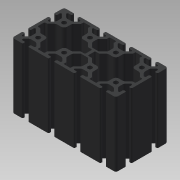
# Autodesk Inventor part: 40-8016
Saved by Autodesk Inventor 2013 (Build 170138000, 138)
## iProperties
Company: 80/20 Inc.
Created: 2014-04-23
Part Number: 40-8016
Material: Generic
Document SubType Name: Modeling
Designer: Ross Bowman
Density: 1 g/cm^3
Engineer: Ross Bowman
Catalog Web Link: 8020.net
Vendor: 80/20 Inc.
Material: 6105-T5 Aluminum
Author: Ross Bowman
Keywords: 80/20 , 8020 , T-Slot , Extrusion
Autodesk Inventor part; units mm, degrees
ref_plane "YZ Plane" through (0, 0, 0) normal (1, 0, 0) x (0, 1, 0)
ref_plane "XZ Plane" through (0, 0, 0) normal (0, 1, 0) x (-1, 0, 0)
ref_plane "XY Plane" through (0, 0, 0) normal (0, 0, 1) x (1, 0, 0)
sketch "Sketch1" plane through (0, 0, 0) normal (0, 0, 1) x (1, 0, 0)
  circle A0 centre (-19.8932, -20) radius 3.4
  circle A1 centre (-59.9459, -20) radius 3.4
  circle A2 centre (-59.9233, 20) radius 3.4
  line L0 (-29.0146, 25.9413) -> (-34.3182, 31.245)
  arc A3 (-27.6247, 22.586) -> (-29.0146, 25.9413) centre (-32.3699, 22.586) ccw
  line L1 (-27.6247, 16.9863) -> (-27.6247, 22.586)
  arc A4 (-27.6247, 16.9863) -> (-22.8702, 12.2331) centre (-22.8715, 16.9863) ccw
  line L2 (-17.2771, 12.2347) -> (-22.8702, 12.2331)
  arc A5 (-13.9164, 10.8432) -> (-17.2771, 12.2347) centre (-17.2757, 7.4839) ccw
  line L3 (-9.0966, 6.0233) -> (-13.9164, 10.8432)
  arc A6 (-9.0966, 6.0233) -> (-8.1978, 5.651) centre (-8.1978, 6.9221) ccw
  line L4 (-3.674, 5.651) -> (-8.1978, 5.651)
  arc A7 (-2.1487, 4.1257) -> (-3.674, 5.651) centre (-3.674, 4.1257) ccw
  line L5 (-2.1487, -4.1257) -> (-2.1487, 4.1257)
  arc A8 (-3.674, -5.651) -> (-2.1487, -4.1257) centre (-3.674, -4.1257) ccw
  line L6 (-8.1978, -5.651) -> (-3.674, -5.651)
  arc A9 (-8.1978, -5.651) -> (-9.0966, -6.0233) centre (-8.1978, -6.9222) ccw
  line L7 (-13.9968, -10.9236) -> (-9.0966, -6.0233)
  arc A10 (-17.3574, -12.315) -> (-13.9968, -10.9236) centre (-17.3561, -7.5643) ccw
  line L8 (-22.9506, -12.3135) -> (-17.3574, -12.315)
  arc A11 (-22.9506, -12.3135) -> (-27.7051, -17.0667) centre (-22.9519, -17.0667) ccw
  line L9 (-27.7051, -22.6663) -> (-27.7051, -17.0667)
  arc A12 (-29.0949, -26.0217) -> (-27.7051, -22.6663) centre (-32.4503, -22.6663) ccw
  line L10 (-34.3986, -31.3253) -> (-29.0949, -26.0217)
  arc A13 (-34.3986, -31.3253) -> (-34.6217, -31.8641) centre (-33.8598, -31.8641) ccw
  line L11 (-34.6217, -34.9245) -> (-34.6217, -31.8641)
  arc A14 (-35.3538, -35.6864) -> (-34.6217, -34.9245) centre (-36.0076, -34.3255) ccw
  line L12 (-44.518, -35.6864) -> (-35.3538, -35.6864)
  arc A15 (-45.2799, -34.9245) -> (-44.518, -35.6864) centre (-44.518, -34.9245) ccw
  line L13 (-45.2799, -31.8641) -> (-45.2799, -34.9245)
  arc A16 (-45.2799, -31.8641) -> (-45.5031, -31.3253) centre (-46.0418, -31.8641) ccw
  line L14 (-50.8067, -26.0217) -> (-45.5031, -31.3253)
  arc A17 (-52.1965, -22.6663) -> (-50.8067, -26.0217) centre (-47.4513, -22.6663) ccw
  line L15 (-52.1965, -17.0667) -> (-52.1965, -22.6663)
  arc A18 (-52.1965, -17.0667) -> (-56.9511, -12.3135) centre (-56.9498, -17.0667) ccw
  line L16 (-62.5442, -12.315) -> (-56.9511, -12.3135)
  arc A19 (-65.9048, -10.9236) -> (-62.5442, -12.315) centre (-62.5455, -7.5643) ccw
  line L17 (-70.805, -6.0233) -> (-65.9048, -10.9236)
  arc A20 (-70.805, -6.0233) -> (-71.7039, -5.651) centre (-71.7039, -6.9222) ccw
  line L18 (-74.0378, -5.651) -> (-71.7039, -5.651)
  arc A21 (-75.5631, -4.1257) -> (-74.0378, -5.651) centre (-74.0378, -4.1257) ccw
  line L19 (-75.5631, 4.1257) -> (-75.5631, -4.1257)
  arc A22 (-74.0378, 5.651) -> (-75.5631, 4.1257) centre (-74.0378, 4.1257) ccw
  line L20 (-71.7842, 5.651) -> (-74.0378, 5.651)
  arc A23 (-71.7842, 5.651) -> (-70.8854, 6.0233) centre (-71.7842, 6.9221) ccw
  line L21 (-66.0655, 10.8433) -> (-70.8854, 6.0233)
  arc A24 (-62.7049, 12.2347) -> (-66.0655, 10.8433) centre (-62.7062, 7.484) ccw
  line L22 (-56.9006, 12.2331) -> (-62.7049, 12.2347)
  arc A25 (-56.9006, 12.2331) -> (-52.146, 16.9863) centre (-56.8993, 16.9863) ccw
  line L23 (-52.146, 22.586) -> (-52.146, 16.9863)
  arc A26 (-50.7562, 25.9413) -> (-52.146, 22.586) centre (-47.4008, 22.586) ccw
  line L24 (-45.4526, 31.245) -> (-50.7562, 25.9413)
  arc A27 (-45.4526, 31.245) -> (-45.2294, 31.7837) centre (-45.9913, 31.7837) ccw
  line L25 (-45.2294, 34.8441) -> (-45.2294, 31.7837)
  arc A28 (-44.4675, 35.606) -> (-45.2294, 34.8441) centre (-44.4675, 34.8441) ccw
  line L26 (-35.3033, 35.606) -> (-44.4675, 35.606)
  arc A29 (-34.5414, 34.8441) -> (-35.3033, 35.606) centre (-35.3033, 34.8441) ccw
  line L27 (-34.5414, 31.7837) -> (-34.5414, 34.8441)
  arc A30 (-34.5414, 31.7837) -> (-34.3182, 31.245) centre (-33.7795, 31.7837) ccw
  circle A31 centre (-19.8932, 20) radius 3.4
  line L28 (5.555, 8.5685) -> (10.7909, 13.8044)
  arc A32 (5.0162, 8.3454) -> (5.555, 8.5685) centre (5.0162, 9.1073) ccw
  line L29 (-4.9936, 8.3454) -> (5.0162, 8.3454)
  arc A33 (-5.5324, 8.5685) -> (-4.9936, 8.3454) centre (-4.9936, 9.1073) ccw
  line L30 (-10.7682, 13.8044) -> (-5.5324, 8.5685)
  arc A34 (-12.1593, 17.1626) -> (-10.7682, 13.8044) centre (-7.4101, 17.1626) ccw
  line L31 (-12.1593, 22.4857) -> (-12.1593, 17.1626)
  arc A35 (-10.7682, 25.8439) -> (-12.1593, 22.4857) centre (-7.4101, 22.4857) ccw
  line L32 (-5.4618, 31.1504) -> (-10.7682, 25.8439)
  arc A36 (-5.4618, 31.1504) -> (-5.2386, 31.6891) centre (-6.0005, 31.6891) ccw
  line L33 (-5.2386, 34.7439) -> (-5.2386, 31.6891)
  arc A37 (-4.4767, 35.5058) -> (-5.2386, 34.7439) centre (-4.4767, 34.7439) ccw
  line L34 (4.4993, 35.5058) -> (-4.4767, 35.5058)
  arc A38 (5.2612, 34.7439) -> (4.4993, 35.5058) centre (4.4993, 34.7439) ccw
  line L35 (5.2612, 31.6891) -> (5.2612, 34.7439)
  arc A39 (5.2612, 31.6891) -> (5.4844, 31.1504) centre (6.0231, 31.6891) ccw
  line L36 (10.7909, 25.8439) -> (5.4844, 31.1504)
  arc A40 (12.1819, 22.4857) -> (10.7909, 25.8439) centre (7.4327, 22.4857) ccw
  line L37 (12.1819, 17.1626) -> (12.1819, 22.4857)
  arc A41 (10.7909, 13.8044) -> (12.1819, 17.1626) centre (7.4327, 17.1626) ccw
  circle A42 centre (19.9158, 20) radius 3.4
  circle A43 centre (59.9459, 20) radius 3.4
  circle A44 centre (59.9685, -20) radius 3.4
  circle A45 centre (19.9158, -20) radius 3.4
  line L38 (5.3117, -34.8242) -> (5.3117, -31.7695)
  arc A46 (4.5498, -35.5861) -> (5.3117, -34.8242) centre (4.5498, -34.8242) ccw
  line L39 (-4.5272, -35.5861) -> (4.5498, -35.5861)
  arc A47 (-5.2891, -34.8242) -> (-4.5272, -35.5861) centre (-4.5272, -34.8242) ccw
  line L40 (-5.2891, -31.7695) -> (-5.2891, -34.8242)
  arc A48 (-5.2891, -31.7695) -> (-5.5123, -31.2307) centre (-6.051, -31.7695) ccw
  line L41 (-10.8187, -25.9243) -> (-5.5123, -31.2307)
  arc A49 (-12.2098, -22.5661) -> (-10.8187, -25.9243) centre (-7.4606, -22.5661) ccw
  line L42 (-12.2098, -17.243) -> (-12.2098, -22.5661)
  arc A50 (-10.8187, -13.8848) -> (-12.2098, -17.243) centre (-7.4606, -17.243) ccw
  line L43 (-5.5829, -8.6489) -> (-10.8187, -13.8848)
  arc A51 (-5.0441, -8.4257) -> (-5.5829, -8.6489) centre (-5.0441, -9.1876) ccw
  line L44 (5.0667, -8.4257) -> (-5.0441, -8.4257)
  arc A52 (5.6055, -8.6489) -> (5.0667, -8.4257) centre (5.0667, -9.1876) ccw
  line L45 (10.8414, -13.8848) -> (5.6055, -8.6489)
  arc A53 (12.2324, -17.243) -> (10.8414, -13.8848) centre (7.4832, -17.243) ccw
  line L46 (12.2324, -22.5661) -> (12.2324, -17.243)
  arc A54 (10.8414, -25.9243) -> (12.2324, -22.5661) centre (7.4832, -22.5661) ccw
  line L47 (5.5349, -31.2307) -> (10.8414, -25.9243)
  arc A55 (5.5349, -31.2307) -> (5.3117, -31.7695) centre (6.0736, -31.7695) ccw
  line L48 (52.1687, 16.9863) -> (52.1687, 22.586)
  arc A56 (52.1687, 16.9863) -> (56.9232, 12.2331) centre (56.9219, 16.9863) ccw
  line L49 (62.7275, 12.2347) -> (56.9232, 12.2331)
  arc A57 (66.0881, 10.8433) -> (62.7275, 12.2347) centre (62.7288, 7.484) ccw
  line L50 (70.908, 6.0233) -> (66.0881, 10.8433)
  arc A58 (70.908, 6.0233) -> (71.8068, 5.651) centre (71.8068, 6.9221) ccw
  line L51 (74.0604, 5.651) -> (71.8068, 5.651)
  arc A59 (75.5857, 4.1257) -> (74.0604, 5.651) centre (74.0604, 4.1257) ccw
  line L52 (75.5857, -4.1257) -> (75.5857, 4.1257)
  arc A60 (74.0604, -5.651) -> (75.5857, -4.1257) centre (74.0604, -4.1257) ccw
  line L53 (71.7265, -5.651) -> (74.0604, -5.651)
  arc A61 (71.7265, -5.651) -> (70.8277, -6.0233) centre (71.7265, -6.9222) ccw
  line L54 (65.9275, -10.9236) -> (70.8277, -6.0233)
  arc A62 (62.5668, -12.315) -> (65.9275, -10.9236) centre (62.5682, -7.5643) ccw
  line L55 (56.9737, -12.3135) -> (62.5668, -12.315)
  arc A63 (56.9737, -12.3135) -> (52.2192, -17.0667) centre (56.9724, -17.0667) ccw
  line L56 (52.2192, -22.6663) -> (52.2192, -17.0667)
  arc A64 (50.8293, -26.0217) -> (52.2192, -22.6663) centre (47.474, -22.6663) ccw
  line L57 (45.5257, -31.3253) -> (50.8293, -26.0217)
  arc A65 (45.5257, -31.3253) -> (45.3025, -31.8641) centre (46.0644, -31.8641) ccw
  line L58 (45.3025, -34.9245) -> (45.3025, -31.8641)
  arc A66 (44.5406, -35.6864) -> (45.3025, -34.9245) centre (44.5406, -34.9245) ccw
  line L59 (35.3764, -35.6864) -> (44.5406, -35.6864)
  arc A67 (34.6443, -34.9245) -> (35.3764, -35.6864) centre (36.0302, -34.3255) ccw
  line L60 (34.6443, -31.8641) -> (34.6443, -34.9245)
  arc A68 (34.6443, -31.8641) -> (34.4212, -31.3253) centre (33.8824, -31.8641) ccw
  line L61 (29.1175, -26.0217) -> (34.4212, -31.3253)
  arc A69 (27.7277, -22.6663) -> (29.1175, -26.0217) centre (32.4729, -22.6663) ccw
  line L62 (27.7277, -17.0667) -> (27.7277, -22.6663)
  arc A70 (27.7277, -17.0667) -> (22.9732, -12.3135) centre (22.9745, -17.0667) ccw
  line L63 (17.38, -12.315) -> (22.9732, -12.3135)
  arc A71 (14.0194, -10.9236) -> (17.38, -12.315) centre (17.3787, -7.5643) ccw
  line L64 (9.1192, -6.0233) -> (14.0194, -10.9236)
  arc A72 (9.1192, -6.0233) -> (8.2204, -5.651) centre (8.2204, -6.9222) ccw
  line L65 (3.6966, -5.651) -> (8.2204, -5.651)
  arc A73 (2.1713, -4.1257) -> (3.6966, -5.651) centre (3.6966, -4.1257) ccw
  line L66 (2.1713, 4.1257) -> (2.1713, -4.1257)
  arc A74 (3.6966, 5.651) -> (2.1713, 4.1257) centre (3.6966, 4.1257) ccw
  line L67 (8.2204, 5.651) -> (3.6966, 5.651)
  arc A75 (8.2204, 5.651) -> (9.1192, 6.0233) centre (8.2204, 6.9221) ccw
  line L68 (13.9391, 10.8432) -> (9.1192, 6.0233)
  arc A76 (17.2997, 12.2347) -> (13.9391, 10.8432) centre (17.2984, 7.4839) ccw
  line L69 (22.8928, 12.2331) -> (17.2997, 12.2347)
  arc A77 (22.8928, 12.2331) -> (27.6473, 16.9863) centre (22.8941, 16.9863) ccw
  line L70 (27.6473, 22.586) -> (27.6473, 16.9863)
  arc A78 (29.0372, 25.9413) -> (27.6473, 22.586) centre (32.3926, 22.586) ccw
  line L71 (34.3408, 31.245) -> (29.0372, 25.9413)
  arc A79 (34.3408, 31.245) -> (34.564, 31.7837) centre (33.8021, 31.7837) ccw
  line L72 (34.564, 34.8441) -> (34.564, 31.7837)
  arc A80 (35.3259, 35.606) -> (34.564, 34.8441) centre (35.3259, 34.8441) ccw
  line L73 (44.4901, 35.606) -> (35.3259, 35.606)
  arc A81 (45.252, 34.8441) -> (44.4901, 35.606) centre (44.4901, 34.8441) ccw
  line L74 (45.252, 31.7837) -> (45.252, 34.8441)
  arc A82 (45.252, 31.7837) -> (45.4752, 31.245) centre (46.0139, 31.7837) ccw
  line L75 (50.7788, 25.9413) -> (45.4752, 31.245)
  arc A83 (52.1687, 22.586) -> (50.7788, 25.9413) centre (47.4235, 22.586) ccw
  arc A84 (-14.2586, 40) -> (-15.8332, 38.4254) centre (-14.2586, 38.4254) ccw
  line L76 (-15.8332, 38.4254) -> (-15.8332, 37)
  arc A85 (-15.8332, 37) -> (-14.1726, 35.3394) centre (-14.1726, 37) ccw
  line L77 (-14.1726, 35.3394) -> (-11.0899, 35.3394)
  arc A86 (-9.5661, 33.8156) -> (-11.0899, 35.3394) centre (-11.0899, 33.8156) ccw
  line L78 (-9.5661, 33.8156) -> (-9.5661, 33.6019)
  arc A87 (-9.7892, 33.0632) -> (-9.5661, 33.6019) centre (-10.328, 33.6019) ccw
  line L79 (-9.7892, 33.0632) -> (-13.778, 29.0744)
  arc A88 (-17.1361, 27.6834) -> (-13.778, 29.0744) centre (-17.1361, 32.4326) ccw
  line L80 (-17.1361, 27.6834) -> (-22.6502, 27.6834)
  arc A89 (-26.0084, 29.0744) -> (-22.6502, 27.6834) centre (-22.6502, 32.4326) ccw
  line L81 (-26.0084, 29.0744) -> (-29.9972, 33.0632)
  arc A90 (-30.2203, 33.6019) -> (-29.9972, 33.0632) centre (-29.4584, 33.6019) ccw
  line L82 (-30.2203, 33.6019) -> (-30.2203, 33.8156)
  arc A91 (-28.6965, 35.3394) -> (-30.2203, 33.8156) centre (-28.6965, 33.8156) ccw
  line L83 (-28.6965, 35.3394) -> (-25.6138, 35.3394)
  arc A92 (-25.6138, 35.3394) -> (-23.9532, 37) centre (-25.6138, 37) ccw
  line L84 (-23.9532, 37) -> (-23.9532, 38.4254)
  arc A93 (-23.9532, 38.4254) -> (-25.5278, 40) centre (-25.5278, 38.4254) ccw
  line L85 (-25.5278, 40) -> (-54.2696, 40)
  arc A94 (-54.2696, 40) -> (-55.8884, 38.3811) centre (-54.2696, 38.3811) ccw
  line L86 (-55.8884, 38.3811) -> (-55.8884, 37.2546)
  arc A95 (-55.8884, 37.2546) -> (-54.3138, 35.68) centre (-54.3138, 37.2546) ccw
  line L87 (-54.3138, 35.68) -> (-51.1219, 35.68)
  arc A96 (-49.5981, 34.1562) -> (-51.1219, 35.68) centre (-51.1219, 34.1562) ccw
  line L88 (-49.5981, 34.1562) -> (-49.5981, 33.5244)
  arc A97 (-49.8212, 32.9857) -> (-49.5981, 33.5244) centre (-50.36, 33.5244) ccw
  line L89 (-49.8212, 32.9857) -> (-53.76, 29.0469)
  arc A98 (-57.0117, 27.7) -> (-53.76, 29.0469) centre (-57.0117, 32.2986) ccw
  line L90 (-57.0117, 27.7) -> (-62.7039, 27.7)
  arc A99 (-65.9556, 29.0469) -> (-62.7039, 27.7) centre (-62.7039, 32.2986) ccw
  line L91 (-65.9556, 29.0469) -> (-69.9449, 33.0362)
  arc A100 (-70.1681, 33.5749) -> (-69.9449, 33.0362) centre (-69.4062, 33.5749) ccw
  line L92 (-70.1681, 33.5749) -> (-70.1681, 34.1562)
  arc A101 (-68.6443, 35.68) -> (-70.1681, 34.1562) centre (-68.6443, 34.1562) ccw
  line L93 (-68.6443, 35.68) -> (-65.4523, 35.68)
  arc A102 (-65.4523, 35.68) -> (-63.8777, 37.2546) centre (-65.4523, 37.2546) ccw
  line L94 (-63.8777, 37.2546) -> (-63.8777, 38.3811)
  arc A103 (-63.8777, 38.3811) -> (-65.4966, 40) centre (-65.4966, 38.3811) ccw
  line L95 (-65.4966, 40) -> (-76.7085, 40)
  arc A104 (-76.7085, 40) -> (-79.8819, 36.9125) centre (-76.7085, 36.8254) ccw
  line L96 (-79.8819, 36.9125) -> (-79.9887, 33.0204)
  line L97 (-79.9887, 33.0204) -> (-79.9887, 25.6135)
  arc A105 (-79.9887, 25.6135) -> (-78.3698, 23.9947) centre (-78.3698, 25.6135) ccw
  line L98 (-78.3698, 23.9947) -> (-77.1377, 23.9947)
  arc A106 (-77.1377, 23.9947) -> (-75.5631, 25.5693) centre (-77.1377, 25.5693) ccw
  line L99 (-75.5631, 25.5693) -> (-75.5631, 28.7612)
  arc A107 (-74.0393, 30.285) -> (-75.5631, 28.7612) centre (-74.0393, 28.7612) ccw
  line L100 (-74.0393, 30.285) -> (-73.5384, 30.285)
  arc A108 (-72.9996, 30.0618) -> (-73.5384, 30.285) centre (-73.5384, 29.5231) ccw
  line L101 (-72.9996, 30.0618) -> (-69.0356, 26.0978)
  arc A109 (-67.6887, 22.8461) -> (-69.0356, 26.0978) centre (-72.2873, 22.8461) ccw
  line L102 (-67.6887, 22.8461) -> (-67.6887, 17.1539)
  arc A110 (-69.0356, 13.9022) -> (-67.6887, 17.1539) centre (-72.2873, 17.1539) ccw
  line L103 (-69.0356, 13.9022) -> (-72.9996, 9.9382)
  arc A111 (-73.5384, 9.715) -> (-72.9996, 9.9382) centre (-73.5384, 10.4769) ccw
  line L104 (-73.5384, 9.715) -> (-74.0393, 9.715)
  arc A112 (-75.5631, 11.2388) -> (-74.0393, 9.715) centre (-74.0393, 11.2388) ccw
  line L105 (-75.5631, 11.2388) -> (-75.5631, 14.4307)
  arc A113 (-75.5631, 14.4307) -> (-77.1377, 16.0053) centre (-77.1377, 14.4307) ccw
  line L106 (-77.1377, 16.0053) -> (-78.3698, 16.0053)
  arc A114 (-78.3698, 16.0053) -> (-79.9887, 14.3865) centre (-78.3698, 14.3865) ccw
  line L107 (-79.9887, 14.3865) -> (-79.9887, -14.3865)
  arc A115 (-79.9887, -14.3865) -> (-78.3698, -16.0053) centre (-78.3698, -14.3865) ccw
  line L108 (-78.3698, -16.0053) -> (-77.2433, -16.0053)
  arc A116 (-77.2433, -16.0053) -> (-75.6687, -14.4307) centre (-77.2433, -14.4307) ccw
  line L109 (-75.6687, -14.4307) -> (-75.6687, -11.2388)
  arc A117 (-74.1449, -9.715) -> (-75.6687, -11.2388) centre (-74.1449, -11.2388) ccw
  line L110 (-74.1449, -9.715) -> (-73.644, -9.715)
  arc A118 (-73.1052, -9.9382) -> (-73.644, -9.715) centre (-73.644, -10.4769) ccw
  line L111 (-73.1052, -9.9382) -> (-69.1159, -13.9275)
  arc A119 (-67.6887, -17.1792) -> (-69.1159, -13.9275) centre (-72.2866, -17.2582) ccw
  line L112 (-67.6887, -17.1792) -> (-67.6887, -22.8209)
  arc A120 (-69.0356, -26.0726) -> (-67.6887, -22.8209) centre (-72.2873, -22.8209) ccw
  line L113 (-69.0356, -26.0726) -> (-73.0249, -30.0618)
  arc A121 (-73.644, -30.285) -> (-73.0249, -30.0618) centre (-73.5675, -29.527) ccw
  line L114 (-73.644, -30.285) -> (-74.1449, -30.285)
  arc A122 (-75.6687, -28.7612) -> (-74.1449, -30.285) centre (-74.1449, -28.7612) ccw
  line L115 (-75.6687, -28.7612) -> (-75.6687, -25.5693)
  arc A123 (-75.6687, -25.5693) -> (-77.2433, -23.9947) centre (-77.2433, -25.5693) ccw
  line L116 (-77.2433, -23.9947) -> (-78.3698, -23.9947)
  arc A124 (-78.3698, -23.9947) -> (-79.9887, -25.6135) centre (-78.3698, -25.6135) ccw
  line L117 (-79.9887, -25.6135) -> (-79.9887, -36.8254)
  arc A125 (-79.9887, -36.8254) -> (-76.8141, -40) centre (-76.8141, -36.8254) ccw
  line L118 (-76.8141, -40) -> (-65.4966, -40)
  arc A126 (-65.4966, -40) -> (-63.8777, -38.3811) centre (-65.4966, -38.3811) ccw
  line L119 (-63.8777, -38.3811) -> (-63.8777, -37.2546)
  arc A127 (-63.8777, -37.2546) -> (-65.4523, -35.68) centre (-65.4523, -37.2546) ccw
  line L120 (-65.4523, -35.68) -> (-68.6443, -35.68)
  arc A128 (-70.1681, -34.1562) -> (-68.6443, -35.68) centre (-68.6443, -34.1562) ccw
  line L121 (-70.1681, -34.1562) -> (-70.1681, -33.6553)
  arc A129 (-69.9449, -33.1165) -> (-70.1681, -33.6553) centre (-69.4062, -33.6553) ccw
  line L122 (-69.9449, -33.1165) -> (-65.9556, -29.1273)
  arc A130 (-62.7039, -27.7804) -> (-65.9556, -29.1273) centre (-62.7039, -32.3789) ccw
  line L123 (-62.7039, -27.7804) -> (-57.0622, -27.7804)
  arc A131 (-53.8105, -29.1273) -> (-57.0622, -27.7804) centre (-57.0622, -32.3789) ccw
  line L124 (-53.8105, -29.1273) -> (-49.8212, -33.1165)
  arc A132 (-49.5981, -33.6553) -> (-49.8212, -33.1165) centre (-50.36, -33.6553) ccw
  line L125 (-49.5981, -33.6553) -> (-49.5981, -34.1562)
  arc A133 (-51.1219, -35.68) -> (-49.5981, -34.1562) centre (-51.1219, -34.1562) ccw
  line L126 (-51.1219, -35.68) -> (-54.3138, -35.68)
  arc A134 (-54.3138, -35.68) -> (-55.8884, -37.2546) centre (-54.3138, -37.2546) ccw
  line L127 (-55.8884, -37.2546) -> (-55.8884, -38.3811)
  arc A135 (-55.8884, -38.3811) -> (-54.2696, -40) centre (-54.2696, -38.3811) ccw
  line L128 (-54.2696, -40) -> (-25.5278, -40)
  arc A136 (-25.5278, -40) -> (-23.9532, -38.4254) centre (-25.5278, -38.4254) ccw
  line L129 (-23.9532, -38.4254) -> (-23.9532, -37)
  arc A137 (-23.9532, -37) -> (-25.6138, -35.3394) centre (-25.6138, -37) ccw
  line L130 (-25.6138, -35.3394) -> (-28.6965, -35.3394)
  arc A138 (-30.2203, -33.8156) -> (-28.6965, -35.3394) centre (-28.6965, -33.8156) ccw
  line L131 (-30.2203, -33.8156) -> (-30.2203, -33.6019)
  arc A139 (-29.9972, -33.0632) -> (-30.2203, -33.6019) centre (-29.4584, -33.6019) ccw
  line L132 (-29.9972, -33.0632) -> (-26.0084, -29.0745)
  arc A140 (-22.6502, -27.6834) -> (-26.0084, -29.0745) centre (-22.6502, -32.4326) ccw
  line L133 (-22.6502, -27.6834) -> (-17.1361, -27.6834)
  arc A141 (-13.778, -29.0745) -> (-17.1361, -27.6834) centre (-17.1361, -32.4326) ccw
  line L134 (-13.778, -29.0745) -> (-9.7892, -33.0632)
  arc A142 (-9.5661, -33.6019) -> (-9.7892, -33.0632) centre (-10.328, -33.6019) ccw
  line L135 (-9.5661, -33.6019) -> (-9.5661, -33.8156)
  arc A143 (-11.0899, -35.3394) -> (-9.5661, -33.8156) centre (-11.0899, -33.8156) ccw
  line L136 (-11.0899, -35.3394) -> (-14.1726, -35.3394)
  arc A144 (-14.1726, -35.3394) -> (-15.8332, -37) centre (-14.1726, -37) ccw
  line L137 (-15.8332, -37) -> (-15.8332, -38.4254)
  arc A145 (-15.8332, -38.4254) -> (-14.2586, -40) centre (-14.2586, -38.4254) ccw
  line L138 (-14.2586, -40) -> (14.2813, -40)
  arc A146 (14.2813, -40) -> (15.8558, -38.4254) centre (14.2813, -38.4254) ccw
  line L139 (15.8558, -38.4254) -> (15.8558, -37)
  arc A147 (15.8558, -37) -> (14.1952, -35.3394) centre (14.1952, -37) ccw
  line L140 (14.1952, -35.3394) -> (11.1125, -35.3394)
  arc A148 (9.5887, -33.8156) -> (11.1125, -35.3394) centre (11.1125, -33.8156) ccw
  line L141 (9.5887, -33.8156) -> (9.5887, -33.6019)
  arc A149 (9.8118, -33.0632) -> (9.5887, -33.6019) centre (10.3506, -33.6019) ccw
  line L142 (9.8118, -33.0632) -> (13.8006, -29.0745)
  arc A150 (17.1588, -27.6834) -> (13.8006, -29.0745) centre (17.1588, -32.4326) ccw
  line L143 (17.1588, -27.6834) -> (22.6729, -27.6834)
  arc A151 (26.0311, -29.0745) -> (22.6729, -27.6834) centre (22.6729, -32.4326) ccw
  line L144 (26.0311, -29.0745) -> (30.0198, -33.0632)
  arc A152 (30.2429, -33.6019) -> (30.0198, -33.0632) centre (29.481, -33.6019) ccw
  line L145 (30.2429, -33.6019) -> (30.2429, -33.8156)
  arc A153 (28.7191, -35.3394) -> (30.2429, -33.8156) centre (28.7191, -33.8156) ccw
  line L146 (28.7191, -35.3394) -> (25.6364, -35.3394)
  arc A154 (25.6364, -35.3394) -> (23.9758, -37) centre (25.6364, -37) ccw
  line L147 (23.9758, -37) -> (23.9758, -38.4254)
  arc A155 (23.9758, -38.4254) -> (25.5504, -40) centre (25.5504, -38.4254) ccw
  line L148 (25.5504, -40) -> (54.2922, -40)
  arc A156 (54.2922, -40) -> (55.911, -38.3811) centre (54.2922, -38.3811) ccw
  line L149 (55.911, -38.3811) -> (55.911, -37.2546)
  arc A157 (55.911, -37.2546) -> (54.3364, -35.68) centre (54.3364, -37.2546) ccw
  line L150 (54.3364, -35.68) -> (51.1445, -35.68)
  arc A158 (49.6207, -34.1562) -> (51.1445, -35.68) centre (51.1445, -34.1562) ccw
  line L151 (49.6207, -34.1562) -> (49.6207, -33.6553)
  arc A159 (49.8439, -33.1165) -> (49.6207, -33.6553) centre (50.3826, -33.6553) ccw
  line L152 (49.8439, -33.1165) -> (53.8332, -29.1273)
  arc A160 (57.0849, -27.7804) -> (53.8332, -29.1273) centre (57.0849, -32.3789) ccw
  line L153 (57.0849, -27.7804) -> (62.7266, -27.7804)
  arc A161 (65.9783, -29.1273) -> (62.7266, -27.7804) centre (62.7266, -32.3789) ccw
  line L154 (65.9783, -29.1273) -> (69.9675, -33.1165)
  arc A162 (70.1907, -33.6553) -> (69.9675, -33.1165) centre (69.4288, -33.6553) ccw
  line L155 (70.1907, -33.6553) -> (70.1907, -34.1562)
  arc A163 (68.6669, -35.68) -> (70.1907, -34.1562) centre (68.6669, -34.1562) ccw
  line L156 (68.6669, -35.68) -> (65.475, -35.68)
  arc A164 (65.475, -35.68) -> (63.9004, -37.2546) centre (65.475, -37.2546) ccw
  line L157 (63.9004, -37.2546) -> (63.9004, -38.3811)
  arc A165 (63.9004, -38.3811) -> (65.5192, -40) centre (65.5192, -38.3811) ccw
  line L158 (65.5192, -40) -> (76.8367, -40)
  arc A166 (76.8367, -40) -> (80.0113, -36.8254) centre (76.8367, -36.8254) ccw
  line L159 (80.0113, -36.8254) -> (80.0113, -25.6135)
  arc A167 (80.0113, -25.6135) -> (78.3925, -23.9947) centre (78.3925, -25.6135) ccw
  line L160 (78.3925, -23.9947) -> (77.2659, -23.9947)
  arc A168 (77.2659, -23.9947) -> (75.6913, -25.5693) centre (77.2659, -25.5693) ccw
  line L161 (75.6913, -25.5693) -> (75.6913, -28.7612)
  arc A169 (74.1675, -30.285) -> (75.6913, -28.7612) centre (74.1675, -28.7612) ccw
  line L162 (74.1675, -30.285) -> (73.6666, -30.285)
  arc A170 (73.0475, -30.0618) -> (73.6666, -30.285) centre (73.5901, -29.527) ccw
  line L163 (73.0475, -30.0618) -> (69.0582, -26.0726)
  arc A171 (67.7113, -22.8209) -> (69.0582, -26.0726) centre (72.3099, -22.8209) ccw
  line L164 (67.7113, -22.8209) -> (67.7113, -17.1792)
  arc A172 (69.1386, -13.9275) -> (67.7113, -17.1792) centre (72.3092, -17.2582) ccw
  line L165 (69.1386, -13.9275) -> (73.1279, -9.9382)
  arc A173 (73.6666, -9.715) -> (73.1279, -9.9382) centre (73.6666, -10.4769) ccw
  line L166 (73.6666, -9.715) -> (74.1675, -9.715)
  arc A174 (75.6913, -11.2388) -> (74.1675, -9.715) centre (74.1675, -11.2388) ccw
  line L167 (75.6913, -11.2388) -> (75.6913, -14.4307)
  arc A175 (75.6913, -14.4307) -> (77.2659, -16.0053) centre (77.2659, -14.4307) ccw
  line L168 (77.2659, -16.0053) -> (78.3925, -16.0053)
  arc A176 (78.3925, -16.0053) -> (80.0113, -14.3865) centre (78.3925, -14.3865) ccw
  line L169 (80.0113, -14.3865) -> (80.0113, 14.3865)
  arc A177 (80.0113, 14.3865) -> (78.3925, 16.0053) centre (78.3925, 14.3865) ccw
  line L170 (78.3925, 16.0053) -> (77.1603, 16.0053)
  arc A178 (77.1603, 16.0053) -> (75.5857, 14.4307) centre (77.1603, 14.4307) ccw
  line L171 (75.5857, 14.4307) -> (75.5857, 11.2388)
  arc A179 (74.0619, 9.715) -> (75.5857, 11.2388) centre (74.0619, 11.2388) ccw
  line L172 (74.0619, 9.715) -> (73.561, 9.715)
  arc A180 (73.0222, 9.9382) -> (73.561, 9.715) centre (73.561, 10.4769) ccw
  line L173 (73.0222, 9.9382) -> (69.0582, 13.9022)
  arc A181 (67.7113, 17.1539) -> (69.0582, 13.9022) centre (72.3099, 17.1539) ccw
  line L174 (67.7113, 17.1539) -> (67.7113, 22.8461)
  arc A182 (69.0582, 26.0978) -> (67.7113, 22.8461) centre (72.3099, 22.8461) ccw
  line L175 (69.0582, 26.0978) -> (73.0222, 30.0618)
  arc A183 (73.561, 30.285) -> (73.0222, 30.0618) centre (73.561, 29.5231) ccw
  line L176 (73.561, 30.285) -> (74.0619, 30.285)
  arc A184 (75.5857, 28.7612) -> (74.0619, 30.285) centre (74.0619, 28.7612) ccw
  line L177 (75.5857, 28.7612) -> (75.5857, 25.5693)
  arc A185 (75.5857, 25.5693) -> (77.1603, 23.9947) centre (77.1603, 25.5693) ccw
  line L178 (77.1603, 23.9947) -> (78.3925, 23.9947)
  arc A186 (78.3925, 23.9947) -> (80.0113, 25.6135) centre (78.3925, 25.6135) ccw
  line L179 (80.0113, 25.6135) -> (80.0113, 33.0204)
  line L180 (80.0113, 33.0204) -> (79.9045, 36.9125)
  arc A187 (79.9045, 36.9125) -> (76.7311, 40) centre (76.7311, 36.8254) ccw
  line L181 (76.7311, 40) -> (65.5192, 40)
  arc A188 (65.5192, 40) -> (63.9004, 38.3811) centre (65.5192, 38.3811) ccw
  line L182 (63.9004, 38.3811) -> (63.9004, 37.2546)
  arc A189 (63.9004, 37.2546) -> (65.475, 35.68) centre (65.475, 37.2546) ccw
  line L183 (65.475, 35.68) -> (68.6669, 35.68)
  arc A190 (70.1907, 34.1562) -> (68.6669, 35.68) centre (68.6669, 34.1562) ccw
  line L184 (70.1907, 34.1562) -> (70.1907, 33.5749)
  arc A191 (69.9675, 33.0362) -> (70.1907, 33.5749) centre (69.4288, 33.5749) ccw
  line L185 (69.9675, 33.0362) -> (65.9783, 29.0469)
  arc A192 (62.7266, 27.7) -> (65.9783, 29.0469) centre (62.7266, 32.2986) ccw
  line L186 (62.7266, 27.7) -> (57.0344, 27.7)
  arc A193 (53.7827, 29.0469) -> (57.0344, 27.7) centre (57.0344, 32.2986) ccw
  line L187 (53.7827, 29.0469) -> (49.8439, 32.9857)
  arc A194 (49.6207, 33.5244) -> (49.8439, 32.9857) centre (50.3826, 33.5244) ccw
  line L188 (49.6207, 33.5244) -> (49.6207, 34.1562)
  arc A195 (51.1445, 35.68) -> (49.6207, 34.1562) centre (51.1445, 34.1562) ccw
  line L189 (51.1445, 35.68) -> (54.3364, 35.68)
  arc A196 (54.3364, 35.68) -> (55.911, 37.2546) centre (54.3364, 37.2546) ccw
  line L190 (55.911, 37.2546) -> (55.911, 38.3811)
  arc A197 (55.911, 38.3811) -> (54.2922, 40) centre (54.2922, 38.3811) ccw
  line L191 (54.2922, 40) -> (25.5504, 40)
  arc A198 (25.5504, 40) -> (23.9758, 38.4254) centre (25.5504, 38.4254) ccw
  line L192 (23.9758, 38.4254) -> (23.9758, 37)
  arc A199 (23.9758, 37) -> (25.6364, 35.3394) centre (25.6364, 37) ccw
  line L193 (25.6364, 35.3394) -> (28.7191, 35.3394)
  arc A200 (30.2429, 33.8156) -> (28.7191, 35.3394) centre (28.7191, 33.8156) ccw
  line L194 (30.2429, 33.8156) -> (30.2429, 33.6019)
  arc A201 (30.0198, 33.0632) -> (30.2429, 33.6019) centre (29.481, 33.6019) ccw
  line L195 (30.0198, 33.0632) -> (26.0311, 29.0744)
  arc A202 (22.6729, 27.6834) -> (26.0311, 29.0744) centre (22.6729, 32.4326) ccw
  line L196 (22.6729, 27.6834) -> (17.1588, 27.6834)
  arc A203 (13.8006, 29.0744) -> (17.1588, 27.6834) centre (17.1588, 32.4326) ccw
  line L197 (13.8006, 29.0744) -> (9.8118, 33.0632)
  arc A204 (9.5887, 33.6019) -> (9.8118, 33.0632) centre (10.3506, 33.6019) ccw
  line L198 (9.5887, 33.6019) -> (9.5887, 33.8156)
  arc A205 (11.1125, 35.3394) -> (9.5887, 33.8156) centre (11.1125, 33.8156) ccw
  line L199 (11.1125, 35.3394) -> (14.1952, 35.3394)
  arc A206 (14.1952, 35.3394) -> (15.8558, 37) centre (14.1952, 37) ccw
  line L200 (15.8558, 37) -> (15.8558, 38.4254)
  arc A207 (15.8558, 38.4254) -> (14.2813, 40) centre (14.2813, 38.4254) ccw
  line L201 (14.2813, 40) -> (-14.2586, 40)
  point P0 (0, 0)
  constraints: 404 end point, 400 point on circle, 208 centre point
extrude "Extrusion1" add sketch "Sketch1" against normal blind 100
body "Solid1"
